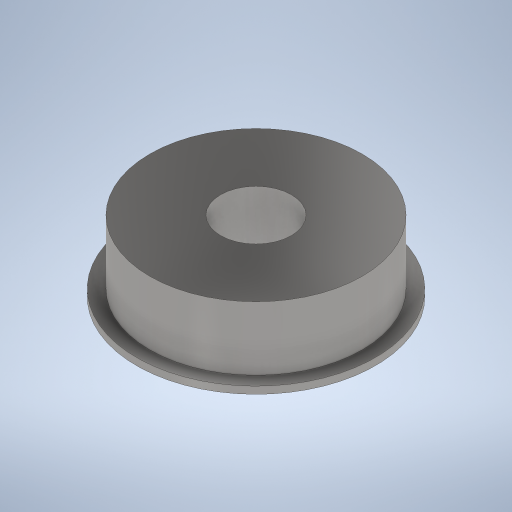
# Autodesk Inventor part: FlangedBearing
Saved by Autodesk Inventor 2024 (Build 280153000, 153)
## iProperties
Created: 2024-01-20
Part Number: FlangedBearing
Material: Generic
Document SubType Name: Modeling
Designer: Irwin
Density: 1 g/cm^3
Appearance: Steel - Polished
Author: Irwin
Autodesk Inventor part; units mm, degrees
ref_plane "YZ Plane" through (0, 0, 0) normal (1, 0, 0) x (0, 1, 0)
ref_plane "XZ Plane" through (0, 0, 0) normal (0, 1, 0) x (-1, 0, 0)
ref_plane "XY Plane" through (0, 0, 0) normal (0, 0, 1) x (1, 0, 0)
sketch "Sketch1" plane through (0, 0, 0) normal (0, 1, 0) x (-1, 0, 0)
  circle A0 centre (0, 0) radius 13.5
  circle A1 centre (0, 0) radius 12
  circle A2 centre (0, 0) radius 4
  dimension "d0" = 27
  dimension "d1" = 24
  dimension "d2" = 8
  constraints: 3 centre point, 3 coincident
  measures "d0" diameter of A0
  measures "d1" diameter of A1
  measures "d2" diameter of A2
extrude "Extrusion1" add sketch "Sketch1" along normal blind 8 contours A1
extrude "Extrusion2" add sketch "Sketch1" along normal blind 0.8 contours A0 | A1 | A2
extrude "Extrusion3" cut sketch "Sketch1" along normal blind 0.8 contours A2
body "Solid1"
